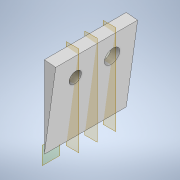
# Autodesk Inventor part: twoPipeCover
Saved by Autodesk Inventor 2021 (Build 250183000, 183)
## iProperties
Created: 2020-07-06
Part Number: twoPipeCover
Material: Generic
Document SubType Name: Modeling
Designer: robst
Density: 1 g/cm^3
Appearance: Default
Author: robst
Autodesk Inventor part; units mm, degrees
ref_plane "YZ Plane" through (0, 0, 0) normal (1, 0, 0) x (0, 1, 0)
ref_plane "XZ Plane" through (0, 0, 0) normal (0, 1, 0) x (-1, 0, 0)
sketch "Sketch1" plane through (0, 0, 0) normal (0, 0, 1) x (1, 0, 0)
  line L0 (0, 0) -> (14.2789, 101.6)
  line L1 (14.2789, 101.6) -> (0, 101.6)
  line L2 (0, 101.6) -> (0, 0)
  dimension "d0" = 101.6
  dimension "d1" = 8
  dimension "d2" = 14.279
  constraints: 6 end point, 1 horizontal, 1 vertical
  measures "d0" distance from line of L0.start L1
  measures "d1" angle of L0 L2
  measures "d2" distance of L0.end L1.end
extrude "Extrusion1" add sketch "Sketch1" along normal mid plane 101.6
ref_plane "Work Plane2" through (0, 0, 42.3872) normal (-1, 0, 0) x (0, 0, 1)
sketch "Sketch6" plane through (0, 0, 42.3872) normal (-1, 0, 0) x (0, 0, 1)
  line L0 (-84.1061, 73.66) -> (0, 73.66) construction
  line L1 (0, 101.6) -> (0, 0) construction
  line L2 (-84.7743, 101.6) -> (0, 101.6) construction
  circle A0 centre (-65.2472, 73.66) radius 9.525
  circle A1 centre (-19.5272, 73.66) radius 7.62
  line L3 (-42.3872, 121.92) -> (-42.3872, -20.32) projected
  point P0 (-42.3872, 0)
  dimension "d18" = 27.94
  dimension "d19" = 19.05
  dimension "d20" = 15.24
  dimension "d21" = 22.86
  dimension "d22" = 22.86
  dimension "d23" = 45.72
  constraints: 3 point on line, 2 centre point, 2 end point, 1 horizontal
  measures "d18" distance between parallel lines of L0 L2
  measures "d19" diameter of A0
  measures "d20" diameter of A1
  measures "d21" distance from line of L3 A0.centre
  measures "d22" distance from line of A1.centre L3
  measures "d23" distance of A1.centre A0.centre
extrude "Extrusion5" cut sketch "Sketch6" against normal through all
ref_plane "Work Plane3" through (0, 0, 22.86) normal (0, 0, 1) x (1, 0, 0)
ref_plane "Work Plane4" through (0, 0, -22.86) normal (0, 0, 1) x (1, 0, 0)
sketch "Sketch9" plane through (0, 0, -50.8) normal (-1, 0, 0) x (0, 0, 1)
  line L0 (0, 101.6) -> (0, 0) construction
  line L1 (0, 38.1) -> (100.9997, 38.1) construction
  line L2 (0, 0) -> (101.6, 0) construction
  spline S0 degree 2 poles (30.4104, 35.6403) (30.4104, 34.6934) (29.6899, 33.2629) (29.093, 32.7895) knots 0 0 0 1 2 2 2
  spline S1 degree 2 poles (29.093, 32.7895) (28.3726, 32.2234) (26.6642, 31.75) (25.3365, 31.75) knots 0 0 0 1 2 2 2
  line L3 (25.3365, 31.75) -> (20.2627, 31.75)
  line L4 (20.2627, 31.75) -> (20.2627, 44.45)
  line L5 (20.2627, 44.45) -> (24.7396, 44.45)
  spline S2 degree 2 poles (24.7396, 44.45) (26.1393, 44.45) (27.5801, 44.2339) (28.2079, 43.8942) knots 0 0 0 1 2 2 2
  spline S3 degree 2 poles (28.2079, 43.8942) (28.8975, 43.534) (29.5664, 42.299) (29.5664, 41.4963) knots 0 0 0 1 2 2 2
  spline S4 degree 2 poles (29.5664, 41.4963) (29.5664, 40.57) (28.6402, 39.1189) (27.8169, 38.7793) knots 0 0 0 1 2 2 2
  line L6 (27.8169, 38.7793) -> (27.8169, 38.7175)
  spline S5 degree 2 poles (27.8169, 38.7175) (29.0004, 38.4705) (30.4104, 36.937) (30.4104, 35.6403) knots 0 0 0 1 2 2 2
  spline S6 degree 2 poles (27.117, 35.6917) (27.117, 36.2887) (26.6436, 36.9576) (26.1702, 37.1326) knots 0 0 0 1 2 2 2
  spline S7 degree 2 poles (26.1702, 37.1326) (25.882, 37.2458) (24.8631, 37.2664) (24.0192, 37.2664) knots 0 0 0 1 2 2 2
  line L7 (24.0192, 37.2664) -> (23.4326, 37.2664)
  line L8 (23.4326, 37.2664) -> (23.4326, 34.0656)
  line L9 (23.4326, 34.0656) -> (23.6075, 34.0656)
  spline S8 degree 2 poles (23.6075, 34.0656) (24.8425, 34.0656) (25.7894, 34.0965) (26.2834, 34.3126) knots 0 0 0 1 2 2 2
  spline S9 degree 2 poles (26.2834, 34.3126) (26.7156, 34.5082) (27.117, 35.2286) (27.117, 35.6917) knots 0 0 0 1 2 2 2
  spline S10 degree 2 poles (26.3246, 40.8685) (26.3246, 41.1772) (26.0055, 41.8256) (25.6762, 41.9697) knots 0 0 0 1 2 2 2
  spline S11 degree 2 poles (25.6762, 41.9697) (25.3674, 42.1138) (24.5029, 42.1344) (23.6487, 42.1344) knots 0 0 0 1 2 2 2
  line L10 (23.6487, 42.1344) -> (23.4326, 42.1344)
  line L11 (23.4326, 42.1344) -> (23.4326, 39.4379)
  line L12 (23.4326, 39.4379) -> (23.834, 39.4379)
  spline S12 degree 2 poles (23.834, 39.4379) (24.647, 39.4379) (25.3057, 39.4688) (25.6556, 39.6335) knots 0 0 0 1 2 2 2
  spline S13 degree 2 poles (25.6556, 39.6335) (26.0364, 39.8187) (26.3246, 40.4465) (26.3246, 40.8685) knots 0 0 0 1 2 2 2
  line L13 (35.9885, 31.75) -> (40.2801, 44.45)
  line L14 (40.2801, 44.45) -> (43.7587, 44.45)
  line L15 (43.7587, 44.45) -> (48.0504, 31.75)
  line L16 (48.0504, 31.75) -> (44.7673, 31.75)
  line L17 (44.7673, 31.75) -> (43.9749, 34.3435)
  line L18 (43.9749, 34.3435) -> (39.9817, 34.3435)
  line L19 (39.9817, 34.3435) -> (39.1789, 31.75)
  line L20 (39.1789, 31.75) -> (35.9885, 31.75)
  line L21 (43.275, 36.6489) -> (41.9783, 40.8479)
  line L22 (41.9783, 40.8479) -> (40.6712, 36.6489)
  line L23 (40.6712, 36.6489) -> (43.275, 36.6489)
  spline S14 degree 2 poles (60.0094, 31.503) (57.1483, 31.503) (53.7932, 34.961) (53.7932, 38.0897) knots 0 0 0 1 2 2 2
  spline S15 degree 2 poles (53.7932, 38.0897) (53.7932, 41.1052) (57.1586, 44.697) (60.0197, 44.697) knots 0 0 0 1 2 2 2
  spline S16 degree 2 poles (60.0197, 44.697) (60.771, 44.697) (61.9854, 44.522) (62.5412, 44.378) knots 0 0 0 1 2 2 2
  spline S17 degree 2 poles (62.5412, 44.378) (62.9734, 44.2442) (63.9923, 43.8016) (64.3113, 43.637) knots 0 0 0 1 2 2 2
  line L24 (64.3113, 43.637) -> (64.3113, 40.6112)
  line L25 (64.3113, 40.6112) -> (63.9923, 40.6112)
  spline S18 degree 2 poles (63.9923, 40.6112) (63.7556, 40.817) (63.0557, 41.3934) (62.6132, 41.6609) knots 0 0 0 1 2 2 2
  spline S19 degree 2 poles (62.6132, 41.6609) (62.1707, 41.9388) (61.1106, 42.3196) (60.524, 42.3196) knots 0 0 0 1 2 2 2
  spline S20 degree 2 poles (60.524, 42.3196) (59.8344, 42.3196) (58.6921, 41.8874) (58.1672, 41.3419) knots 0 0 0 1 2 2 2
  spline S21 degree 2 poles (58.1672, 41.3419) (57.6938, 40.8582) (57.0865, 39.2012) (57.0865, 38.0794) knots 0 0 0 1 2 2 2
  spline S22 degree 2 poles (57.0865, 38.0794) (57.0865, 36.8959) (57.7143, 35.2801) (58.2289, 34.7861) knots 0 0 0 1 2 2 2
  spline S23 degree 2 poles (58.2289, 34.7861) (58.7229, 34.3024) (59.9374, 33.8804) (60.5446, 33.8804) knots 0 0 0 1 2 2 2
  spline S24 degree 2 poles (60.5446, 33.8804) (61.1724, 33.8804) (62.3147, 34.3024) (62.7058, 34.5596) knots 0 0 0 1 2 2 2
  spline S25 degree 2 poles (62.7058, 34.5596) (63.1381, 34.8169) (63.7865, 35.3624) (64.0232, 35.5785) knots 0 0 0 1 2 2 2
  line L26 (64.0232, 35.5785) -> (64.3113, 35.5785)
  line L27 (64.3113, 35.5785) -> (64.3113, 32.5939)
  spline S26 degree 2 poles (64.3113, 32.5939) (63.9614, 32.4293) (63.0455, 32.0176) (62.5515, 31.8735) knots 0 0 0 1 2 2 2
  spline S27 degree 2 poles (62.5515, 31.8735) (61.9545, 31.6882) (60.9151, 31.503) (60.0094, 31.503) knots 0 0 0 1 2 2 2
  line L28 (82.4351, 31.75) -> (78.5757, 31.75)
  line L29 (78.5757, 31.75) -> (75.128, 36.9062)
  line L30 (75.128, 36.9062) -> (74.5002, 36.0417)
  line L31 (74.5002, 36.0417) -> (74.5002, 31.75)
  line L32 (74.5002, 31.75) -> (71.3097, 31.75)
  line L33 (71.3097, 31.75) -> (71.3097, 44.45)
  line L34 (71.3097, 44.45) -> (74.5002, 44.45)
  line L35 (74.5002, 44.45) -> (74.5002, 38.7793)
  line L36 (74.5002, 38.7793) -> (78.5757, 44.45)
  line L37 (78.5757, 44.45) -> (82.2498, 44.45)
  line L38 (82.2498, 44.45) -> (77.7215, 38.5528)
  line L39 (77.7215, 38.5528) -> (82.4351, 31.75)
  point P0 (50.8, 0)
  dimension "d35" = 38.1
  constraints: 2 end point, 2 horizontal, 1 point on line
  measures "d35" distance between parallel lines of L1 L2
extrude "TextforBack" cut sketch "Sketch9" against normal blind 2.54
sketch "Sketch10" plane through (0, 0, 0) normal (0, 0, 1) x (1, 0, 0)
  line L0 (14.2789, 101.6) -> (0, 0) projected
  line L1 (0, 101.6) -> (14.2789, 101.6) projected
  line L2 (0, 0) -> (0, 101.6) projected
  line L3 (0, 101.6) -> (14.1055, 100.3659)
  line L4 (0, 101.6) -> (14.1594, 101.6) construction
  line L5 (14.1055, 100.3659) -> (14.2789, 101.6)
  line L6 (14.2789, 101.6) -> (0, 101.6)
  dimension "d38" = 5
  constraints: 8 end point, 2 collinear, 1 equal length, 1 horizontal, 1 point on line
  measures "d38" angle of L3 L4
extrude "Extrusion8" cut sketch "Sketch10" against normal through all both and the other way through all contours L0 L3 L1
body "Solid1"
